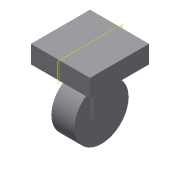
# Autodesk Inventor part: Caster
Saved by Autodesk Inventor 2019 (Build 230136000, 136)
## iProperties
Created: 2019-04-28
Part Number: Caster
Material: 고무
Document SubType Name: Modeling
Designer: hinmo
Mass: 297.093 g
Surface Area: 403.482 cm^2
Volume: 319.454 cm^3
Density: 0.93 g/cm^3
Appearance: 고무 - 검은색
Author: hinmo
Autodesk Inventor part; units mm, degrees
ref_plane "YZ Plane" through (0, 0, 0) normal (1, 0, 0) x (0, 1, 0)
ref_plane "XZ Plane" through (0, 0, 0) normal (0, 1, 0) x (-1, 0, 0)
ref_plane "XY Plane" through (0, 0, 0) normal (0, 0, 1) x (1, 0, 0)
sketch "스케치1" plane through (0, 0, 0) normal (1, 0, 0) x (0, 1, 0)
  line L0 (-12.35, 41) -> (12.35, 41)
  line L1 (12.35, 41) -> (12.35, -41)
  line L2 (12.35, -41) -> (-12.35, -41)
  line L3 (-12.35, -41) -> (-12.35, 41)
  line L4 (-12.35, 41) -> (12.35, -41) construction
  line L5 (12.35, 41) -> (-12.35, -41) construction
  point P0 (0, 0)
  dimension "d0" = 24.7
  dimension "d1" = 82
  constraints: 12 end point, 2 midpoint, 2 parallel, 1 horizontal, 1 perpendicular
  measures "d0" distance of L1.end L2.end
  measures "d1" distance of L0.end L1.end
extrude "돌출1" add sketch "스케치1" along normal blind 82
ref_plane "작업 평면1" through (41, 0, 0) normal (1, 0, 0) x (0, 0, -1)
sketch "스케치2" plane through (41, 0, 0) normal (1, 0, 0) x (0, 0, -1)
  line L0 (-41, 12.35) -> (-41, -12.35) projected
  line L1 (-41, -12.35) -> (41, -12.35) projected
  line L2 (41, -12.35) -> (41, 12.35) projected
  line L3 (41, 12.35) -> (-41, 12.35) projected
  line L4 (0, -12.35) -> (0, -62.35)
  circle A0 centre (0, -62.35) radius 37.5
  point P0 (0, 0)
  dimension "d5" = 50
  dimension "d6" = 75
  constraints: 2 end point, 1 centre point, 1 coincident, 1 midpoint, 1 vertical
  measures "d5" distance of L4.start L4.end
  measures "d6" diameter of A0
extrude "돌출2" add sketch "스케치2" along normal mid plane 32 contours A0
sketch "스케치3" plane through (57, -62.35, 0) normal (1, 0, 0) x (0, 0, -1)
  line L0 (-41, 50) -> (41, 50) projected
  line L1 (0, 50) -> (-15, 50)
  line L2 (-15, 50) -> (-15, 0)
  line L3 (-15, 0) -> (15, 0)
  line L4 (15, 0) -> (15, 50)
  point P0 (0, 62.35)
  dimension "d9" = 15
  dimension "d10" = 50
  dimension "d11" = 30
  constraints: 8 end point, 3 perpendicular, 2 point on line, 1 midpoint
  measures "d9" distance of L1.start L1.end
  measures "d10" distance of L1.end L2.end
  measures "d11" distance of L2.end L3.end
extrude "돌출3" add sketch "스케치3" along normal blind 4
sketch "스케치4" plane through (25, -62.35, 0) normal (-1, 0, 0) x (0, 0, 1)
  line L0 (0, 0) -> (-15, 0)
  line L1 (-15, 0) -> (-15, 50)
  line L2 (41, 50) -> (-41, 50) projected
  line L3 (15, 50) -> (15, 34.3693) projected
  line L4 (15, 50) -> (15, 0)
  line L5 (15, 0) -> (15, 34.3693) projected
  line L6 (-15, 0) -> (15, 0)
  line L7 (15, 50) -> (-15, 50)
  point P0 (0, 62.35)
  constraints: 10 end point, 2 horizontal, 2 point on line, 1 collinear, 1 perpendicular
extrude "돌출4" add sketch "스케치4" along normal blind 4
